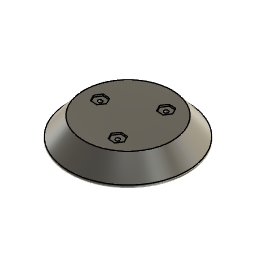
gaseta EMF tapa v7 (Autodesk Fusion 360 design; units mm, degrees)
Autodesk Fusion 360 part; units mm, degrees
sketch "Boceto1" plane through (0, 0, 0) normal (0, 0, 1) x (1, 0, 0)
  circle A0 centre (0, 0) radius 55
  circle A1 centre (-35, 0) radius 2.5
  line L0 (-39.7261, -7.257) -> (-31.0783, -7.7214)
  line L1 (-31.0783, -7.7214) -> (-26.3522, -0.4644)
  line L2 (-26.3522, -0.4644) -> (-30.2739, 7.257)
  line L3 (-30.2739, 7.257) -> (-38.9217, 7.7214)
  line L4 (-38.9217, 7.7214) -> (-43.6478, 0.4644)
  line L5 (-43.6478, 0.4644) -> (-39.7261, -7.257)
  line L6 (13.5783, -22.5895) -> (8.8522, -29.8465)
  line L7 (12.7739, -37.5679) -> (21.4217, -38.0323)
  line L8 (22.2261, -23.0539) -> (13.5783, -22.5895)
  line L9 (26.1478, -30.7753) -> (22.2261, -23.0539)
  circle A2 centre (17.5, -30.3109) radius 2.5
  line L10 (21.4217, -38.0323) -> (26.1478, -30.7753)
  line L11 (8.8522, -29.8465) -> (12.7739, -37.5679)
  line L12 (12.7739, 23.0539) -> (21.4217, 22.5895)
  line L13 (26.1478, 29.8465) -> (22.2261, 37.5679)
  line L14 (8.8522, 30.7753) -> (12.7739, 23.0539)
  line L15 (13.5783, 38.0323) -> (8.8522, 30.7753)
  circle A3 centre (17.5, 30.3109) radius 2.5
  line L16 (22.2261, 37.5679) -> (13.5783, 38.0323)
  line L17 (21.4217, 22.5895) -> (26.1478, 29.8465)
  point P0 (-35, 0)
  point P1 (17.5, -30.3109)
  point P2 (17.5, 30.3109)
  dimension "d1" = 110
  dimension "d30" = 5
  dimension "d31" = 35
  dimension "d32" = 15
  dimension "d34" = 360
  dimension "d37" = 7.257
  constraint coincident A0.centre origin
  constraint coincident P0 A1.centre
  measures "d1" diameter of A0
  measures "d30" diameter of A1
  measures "d31" distance of A0.centre A1.centre
  measures "d32" distance of L2.end L4.end
  measures "d37" vertical distance of P0 L0.start
extrude "Extruir1" add sketch "Boceto1" along normal blind 2 contours A0
sketch "Boceto2" plane through (0, 0, 0) normal (0, 0, -1) x (1, 0, 0)
  circle A0 centre (0, 0) radius 55
  circle A1 centre (0, 0) radius 55
  circle A2 centre (-35, 0) radius 2.5
  circle A3 centre (17.5, 30.3109) radius 2.5
  circle A4 centre (17.5, -30.3109) radius 2.5
  line L0 (8.8522, 29.8465) -> (12.7739, 37.5679)
  line L1 (12.7739, 37.5679) -> (21.4217, 38.0323)
  line L2 (21.4217, 38.0323) -> (26.1478, 30.7753)
  line L3 (26.1478, 30.7753) -> (22.2261, 23.0539)
  line L4 (22.2261, 23.0539) -> (13.5783, 22.5895)
  line L5 (13.5783, 22.5895) -> (8.8522, 29.8465)
  line L6 (-43.6478, -0.4644) -> (-39.7261, 7.257)
  line L7 (-39.7261, 7.257) -> (-31.0783, 7.7214)
  line L8 (-31.0783, 7.7214) -> (-26.3522, 0.4644)
  line L9 (-26.3522, 0.4644) -> (-30.2739, -7.257)
  line L10 (-30.2739, -7.257) -> (-38.9217, -7.7214)
  line L11 (-38.9217, -7.7214) -> (-43.6478, -0.4644)
  line L12 (21.4217, -22.5895) -> (26.1478, -29.8465)
  line L13 (26.1478, -29.8465) -> (22.2261, -37.5679)
  line L14 (22.2261, -37.5679) -> (13.5783, -38.0323)
  line L15 (13.5783, -38.0323) -> (8.8522, -30.7753)
  line L16 (8.8522, -30.7753) -> (12.7739, -23.0539)
  line L17 (12.7739, -23.0539) -> (21.4217, -22.5895)
  circle A5 centre (-35, 0) radius 7.5
  point P0 (17.5, -30.3109)
  point P1 (17.5, 30.3109)
  dimension "d10" = 5
  dimension "d13" = 360
  dimension "d14" = 5
  dimension "d15" = 5
  dimension "d35" = 35
  dimension "d36" = 7.257
  dimension "d47" = 15
  constraint concentric A0 A1
  constraint coincident P1 A3.centre
  constraint coincident P0 A4.centre
  constraint concentric A2 A5
  measures "d10" diameter of A2
  measures "d14" diameter of A3
  measures "d15" diameter of A4
  measures "d35" horizontal distance of A0.centre A2.centre
  measures "d36" vertical distance of A2.centre L9.end
  measures "d47" diameter of A5
extrude "Extruir2" add sketch "Boceto2" along normal blind 2 contours A0 A1 | L0 L1 L2 L3 L4 L5 | L6 L11 A5 | L6 L7 A5 | A5 | L10 L11 A5 | L7 L8 A5 | L9 L10 A5 | L8 L9 A5 | L12 L13 L14 L15 L16 L17
sketch "Boceto3" plane through (0, 0, 0) normal (1, 0, 0) x (0, 1, 0)
  line L0 (55, 2) -> (51.2281, -1.165)
  line L1 (51.2281, -1.165) -> (70.5424, -24.1829)
  line L2 (74.253, -20.9448) -> (55, 2)
  arc A0 (70.5424, -24.1829) -> (74.253, -20.9448) centre (72.3977, -22.5638) ccw
  line L3 (55, 2) -> (81.3501, 2) construction
  line L4 (-55, -2) -> (55, -2)
  dimension "d18" = 50
  dimension "d19" = 30
  dimension "d20" = 4
  dimension "d21" = 55
  dimension "d23" = 20.5638
  dimension "d24" = 2.4624
  constraint perpendicular L0 L1
  constraint parallel L1 L2
  constraint horizontal L3
  measures "d18" angle of L2 L3
  measures "d19" distance of L0 A0.centre
  measures "d20" distance of L0.start L4
  measures "d21" horizontal distance of origin L0.start
  measures "d23" vertical distance of A0.centre L4.end
  measures "d24" radius of A0
revolve "Revolución1" add sketch "Boceto3" angle 360 about axis through (0, 0, 1.75) along (0, 0, 1)
sketch "Boceto4" plane through (0, 0, -2) normal (0, 0, -1) x (1, 0, 0)
  circle A0 centre (0, 0) radius 51.9287
  circle A1 centre (-35, 0) radius 2.5
  line L0 (0, 0) -> (-35, 0)
  circle A2 centre (-35, 0) radius 6
  circle A3 centre (17.5, -30.3109) radius 6
  circle A4 centre (17.5, -30.3109) radius 2.5
  circle A5 centre (17.5, 30.3109) radius 6
  circle A6 centre (17.5, 30.3109) radius 2.5
  point P0 (17.5, -30.3109)
  point P1 (17.5, 30.3109)
  dimension "d40" = 5
  dimension "d41" = 35
  dimension "d42" = 12
  dimension "d44" = 360
  constraint coincident A0.centre L0.start
  constraint horizontal L0
  constraint coincident A1.centre L0.end
  constraint concentric A1 A2
  measures "d40" diameter of A1
  measures "d41" horizontal distance of A0.centre A1.centre
  measures "d42" diameter of A2
extrude "Extruir3" add sketch "Boceto4" along normal blind 20 contours A2 | A3 | A5
